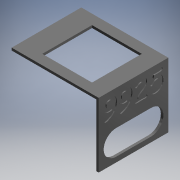
# Autodesk Inventor part: Gen2 Capstone 3D Print 2.0
Saved by Autodesk Inventor 2019 (Build 230136000, 136)
## iProperties
Part Number: Gen2 Capstone 3D Print 2.0
Material: Generic
Document SubType Name: Modeling
Designer: Delta
Appearance: Default
Author: Delta
Autodesk Inventor part; units mm, degrees
ref_plane "YZ Plane" through (0, 0, 0) normal (1, 0, 0) x (0, 1, 0)
ref_plane "XZ Plane" through (0, 0, 0) normal (0, 1, 0) x (-1, 0, 0)
ref_plane "XY Plane" through (0, 0, 0) normal (0, 0, 1) x (1, 0, 0)
sketch "Sketch1" plane through (0, 0, 0) normal (0, 1, 0) x (-1, 0, 0)
  line L0 (0, 0) -> (107.95, 0)
  line L1 (107.95, 0) -> (107.95, -88.9)
  line L2 (107.95, -88.9) -> (0, -88.9)
  line L3 (0, -88.9) -> (0, 0)
  line L4 (81.534, -12.7) -> (18.034, -12.7)
  line L5 (18.034, -12.7) -> (18.034, -76.2)
  line L6 (18.034, -76.2) -> (81.534, -76.2)
  line L7 (81.534, -76.2) -> (81.534, -12.7)
  dimension "d0" = 107.95
  dimension "d1" = 88.9
  dimension "d2" = 63.5
  dimension "d3" = 63.5
  dimension "d4" = 18.034
  dimension "d5" = 12.7
  constraints: 16 end point, 4 parallel, 2 horizontal, 2 perpendicular
  measures "d0" distance of L1.end L2.end
  measures "d1" distance of L0.end L1.end
  measures "d2" distance of L6.end L4.start
  measures "d3" distance of L5.end L6.end
  measures "d4" distance between parallel lines of L3 L5
  measures "d5" distance between parallel lines of L0 L4
extrude "Extrusion1" add sketch "Sketch1" along normal blind 3.175
sketch "Sketch2" plane through (0, 0, 0) normal (1, 0, 0) x (0, 0, -1)
  line L0 (0, 3.175) -> (88.9, 3.175) projected
  line L1 (0, 3.175) -> (88.9, 3.175)
  line L2 (88.9, 3.175) -> (88.9, -79.375)
  line L3 (88.9, -79.375) -> (0, -79.375)
  line L4 (0, -79.375) -> (0, 3.175)
  point P0 (0, 0)
  dimension "d8" = 82.55
  dimension "d9" = 88.9
  dimension "d10" = 88.9
  constraints: 8 end point, 2 parallel, 1 horizontal, 1 perpendicular
  measures "d8" distance of L1.end L2.end
  measures "d9" distance of L0.start L0.end
  measures "d10" distance of L2.end L3.end
extrude "Extrusion2" add sketch "Sketch2" along normal blind 3.175
sketch "Sketch3" plane through (3.175, 0, 0) normal (1, 0, 0) x (0, 0, -1)
  line L0 (4.7988, -3.0029) -> (83.6975, -3.0029) construction
  line L1 (83.6975, -3.0029) -> (83.6975, -35.0341) construction
  line L2 (83.6975, -35.0341) -> (4.7988, -35.0341) construction
  line L3 (4.7988, -35.0341) -> (4.7988, -3.0029) construction
  spline S0 degree 2 poles (17.2249, -18.6506) (16.2825, -18.9793) (14.6827, -19.308) (14.0471, -19.308) knots 0 0 0 1 2 2 2
  spline S1 degree 2 poles (14.0471, -19.308) (10.8913, -19.308) (8.5244, -17.6205) knots 0 0 0 1 1 1
  spline S2 degree 2 poles (8.5244, -17.6205) (5.6316, -15.5386) (5.6316, -11.6814) knots 0 0 0 1 1 1
  spline S3 degree 2 poles (5.6316, -11.6814) (5.6316, -7.2107) (8.5902, -4.9315) knots 0 0 0 1 1 1
  spline S4 degree 2 poles (8.5902, -4.9315) (11.0666, -3.0248) (15.0552, -3.0248) knots 0 0 0 1 1 1
  spline S5 degree 2 poles (15.0552, -3.0248) (18.211, -3.0248) (20.6875, -5.4575) knots 0 0 0 1 1 1
  spline S6 degree 2 poles (20.6875, -5.4575) (23.2735, -7.9996) (23.2954, -11.6157) knots 0 0 0 1 1 1
  spline S7 degree 2 poles (23.2954, -11.6157) (23.3173, -15.5605) (21.7613, -19.2423) knots 0 0 0 1 1 1
  spline S8 degree 2 poles (21.7613, -19.2423) (20.0958, -23.2528) (17.2029, -25.2909) knots 0 0 0 1 1 1
  spline S9 degree 2 poles (17.2029, -25.2909) (15.9976, -26.1456) (13.4116, -27.3291) knots 0 0 0 1 1 1
  spline S10 degree 2 poles (13.4116, -27.3291) (10.453, -28.6659) (9.2257, -28.6659) knots 0 0 0 1 1 1
  spline S11 degree 2 poles (9.2257, -28.6659) (8.3053, -28.6659) (7.6916, -28.0084) knots 0 0 0 1 1 1
  spline S12 degree 2 poles (7.6916, -28.0084) (7.1218, -27.3948) (7.1218, -26.5839) knots 0 0 0 1 1 1
  spline S13 degree 2 poles (7.1218, -26.5839) (7.1218, -25.3128) (8.634, -24.6554) knots 0 0 0 1 1 1
  spline S14 degree 2 poles (8.634, -24.6554) (9.927, -24.239) (11.22, -23.8226) knots 0 0 0 1 1 1
  spline S15 degree 2 poles (11.22, -23.8226) (13.5211, -22.946) (16.151, -20.6887) (17.2249, -18.6506) knots 0 0 0 1 2 2 2
  spline S16 degree 2 poles (14.595, -6.7724) (12.272, -6.7724) (9.9489, -9.0735) (9.927, -11.4185) knots 0 0 0 1 2 2 2
  spline S17 degree 2 poles (9.927, -11.4185) (9.927, -13.3032) (11.3077, -14.3551) knots 0 0 0 1 1 1
  spline S18 degree 2 poles (11.3077, -14.3551) (12.5349, -15.2975) (14.5073, -15.2975) knots 0 0 0 1 1 1
  spline S19 degree 2 poles (14.5073, -15.2975) (15.2963, -15.2975) (17.444, -14.3113) (18.8247, -13.347) knots 0 0 0 1 2 2 2
  spline S20 degree 2 poles (18.8247, -13.347) (18.9781, -12.2512) (18.9781, -11.6157) knots 0 0 0 1 1 1
  spline S21 degree 2 poles (18.9781, -11.6157) (18.9562, -9.972) (17.4878, -8.3503) knots 0 0 0 1 1 1
  spline S22 degree 2 poles (17.4878, -8.3503) (16.0195, -6.7724) (14.595, -6.7724) knots 0 0 0 1 1 1
  spline S23 degree 2 poles (36.883, -18.6506) (35.9406, -18.9793) (34.3408, -19.308) (33.7053, -19.308) knots 0 0 0 1 2 2 2
  spline S24 degree 2 poles (33.7053, -19.308) (30.5494, -19.308) (28.1826, -17.6205) knots 0 0 0 1 1 1
  spline S25 degree 2 poles (28.1826, -17.6205) (25.2897, -15.5386) (25.2897, -11.6814) knots 0 0 0 1 1 1
  spline S26 degree 2 poles (25.2897, -11.6814) (25.2897, -7.2107) (28.2483, -4.9315) knots 0 0 0 1 1 1
  spline S27 degree 2 poles (28.2483, -4.9315) (30.7248, -3.0248) (34.7134, -3.0248) knots 0 0 0 1 1 1
  spline S28 degree 2 poles (34.7134, -3.0248) (37.8692, -3.0248) (40.3456, -5.4575) knots 0 0 0 1 1 1
  spline S29 degree 2 poles (40.3456, -5.4575) (42.9317, -7.9996) (42.9536, -11.6157) knots 0 0 0 1 1 1
  spline S30 degree 2 poles (42.9536, -11.6157) (42.9755, -15.5605) (41.4195, -19.2423) knots 0 0 0 1 1 1
  spline S31 degree 2 poles (41.4195, -19.2423) (39.7539, -23.2528) (36.8611, -25.2909) knots 0 0 0 1 1 1
  spline S32 degree 2 poles (36.8611, -25.2909) (35.6557, -26.1456) (33.0697, -27.3291) knots 0 0 0 1 1 1
  spline S33 degree 2 poles (33.0697, -27.3291) (30.1111, -28.6659) (28.8839, -28.6659) knots 0 0 0 1 1 1
  spline S34 degree 2 poles (28.8839, -28.6659) (27.9634, -28.6659) (27.3498, -28.0084) knots 0 0 0 1 1 1
  spline S35 degree 2 poles (27.3498, -28.0084) (26.78, -27.3948) (26.78, -26.5839) knots 0 0 0 1 1 1
  spline S36 degree 2 poles (26.78, -26.5839) (26.78, -25.3128) (28.2921, -24.6554) knots 0 0 0 1 1 1
  spline S37 degree 2 poles (28.2921, -24.6554) (29.5852, -24.239) (30.8782, -23.8226) knots 0 0 0 1 1 1
  spline S38 degree 2 poles (30.8782, -23.8226) (33.1793, -22.946) (35.8091, -20.6887) (36.883, -18.6506) knots 0 0 0 1 2 2 2
  spline S39 degree 2 poles (34.2532, -6.7724) (31.9301, -6.7724) (29.6071, -9.0735) (29.5852, -11.4185) knots 0 0 0 1 2 2 2
  spline S40 degree 2 poles (29.5852, -11.4185) (29.5852, -13.3032) (30.9658, -14.3551) knots 0 0 0 1 1 1
  spline S41 degree 2 poles (30.9658, -14.3551) (32.1931, -15.2975) (34.1655, -15.2975) knots 0 0 0 1 1 1
  spline S42 degree 2 poles (34.1655, -15.2975) (34.9544, -15.2975) (37.1022, -14.3113) (38.4828, -13.347) knots 0 0 0 1 2 2 2
  spline S43 degree 2 poles (38.4828, -13.347) (38.6362, -12.2512) (38.6362, -11.6157) knots 0 0 0 1 1 1
  spline S44 degree 2 poles (38.6362, -11.6157) (38.6143, -9.972) (37.146, -8.3503) knots 0 0 0 1 1 1
  spline S45 degree 2 poles (37.146, -8.3503) (35.6777, -6.7724) (34.2532, -6.7724) knots 0 0 0 1 1 1
  spline S46 degree 2 poles (59.96, -27.1976) (59.5655, -27.1976) (57.9218, -26.9565) (57.5493, -26.9565) knots 0 0 0 1 2 2 2
  line L4 (57.5493, -26.9565) -> (52.947, -26.9346)
  spline S47 degree 2 poles (52.947, -26.9346) (52.3553, -26.9346) (49.9227, -27.1976) (49.331, -27.1976) knots 0 0 0 1 2 2 2
  spline S48 degree 2 poles (49.331, -27.1976) (49.1557, -27.1976) (48.4982, -27.0661) (48.3229, -27.0661) knots 0 0 0 1 2 2 2
  spline S49 degree 2 poles (48.3229, -27.0661) (46.8984, -27.0661) (46.3943, -25.9265) knots 0 0 0 1 1 1
  spline S50 degree 2 poles (46.3943, -25.9265) (46.0875, -25.2033) (46.0875, -23.6911) knots 0 0 0 1 1 1
  spline S51 degree 2 poles (46.0875, -23.6911) (46.0875, -20.7544) (47.4024, -18.782) knots 0 0 0 1 1 1
  spline S52 degree 2 poles (47.4024, -18.782) (48.3886, -17.2699) (50.6459, -15.7358) knots 0 0 0 1 1 1
  spline S53 degree 2 poles (50.6459, -15.7358) (52.7717, -14.3332) (54.8756, -12.9525) knots 0 0 0 1 1 1
  spline S54 degree 2 poles (54.8756, -12.9525) (57.352, -11.1555) (57.352, -8.8543) knots 0 0 0 1 1 1
  spline S55 degree 2 poles (57.352, -8.8543) (57.352, -8.2626) (55.3796, -7.0792) (54.4373, -7.0792) knots 0 0 0 1 2 2 2
  spline S56 degree 2 poles (54.4373, -7.0792) (52.7717, -7.0792) (49.0461, -10.0597) (48.3448, -10.0597) knots 0 0 0 1 2 2 2
  spline S57 degree 2 poles (48.3448, -10.0597) (47.512, -10.0597) (46.8984, -9.6433) knots 0 0 0 1 1 1
  spline S58 degree 2 poles (46.8984, -9.6433) (46.1094, -9.1392) (46.1094, -8.2407) knots 0 0 0 1 1 1
  spline S59 degree 2 poles (46.1094, -8.2407) (46.1094, -7.2984) (46.8984, -6.5971) knots 0 0 0 1 1 1
  spline S60 degree 2 poles (46.8984, -6.5971) (48.7831, -4.9096) (50.2076, -4.1425) knots 0 0 0 1 1 1
  spline S61 degree 2 poles (50.2076, -4.1425) (52.2457, -3.0248) (54.4373, -3.0248) knots 0 0 0 1 1 1
  spline S62 degree 2 poles (54.4373, -3.0248) (57.1548, -3.0248) (59.3244, -4.4493) knots 0 0 0 1 1 1
  spline S63 degree 2 poles (59.3244, -4.4493) (61.8228, -6.093) (61.8228, -8.7229) knots 0 0 0 1 1 1
  spline S64 degree 2 poles (61.8228, -8.7229) (61.8228, -11.3965) (60.5955, -13.2813) knots 0 0 0 1 1 1
  spline S65 degree 2 poles (60.5955, -13.2813) (59.6531, -14.7715) (57.5712, -16.1741) knots 0 0 0 1 1 1
  spline S66 degree 2 poles (57.5712, -16.1741) (55.6207, -17.4233) (53.6483, -18.6506) knots 0 0 0 1 1 1
  spline S67 degree 2 poles (53.6483, -18.6506) (50.6678, -20.601) (50.4487, -23.0994) knots 0 0 0 1 1 1
  spline S68 degree 2 poles (50.4487, -23.0994) (51.3034, -22.9898) (52.9909, -22.8583) knots 0 0 0 1 1 1
  spline S69 degree 2 poles (52.9909, -22.8583) (56.322, -22.683) (57.7684, -22.683) knots 0 0 0 1 1 1
  spline S70 degree 2 poles (57.7684, -22.683) (59.1272, -22.683) (60.4421, -23.2528) knots 0 0 0 1 1 1
  spline S71 degree 2 poles (60.4421, -23.2528) (62.0638, -23.976) (62.0638, -25.1156) knots 0 0 0 1 1 1
  spline S72 degree 2 poles (62.0638, -25.1156) (62.0638, -25.9265) (61.494, -26.5401) knots 0 0 0 1 1 1
  spline S73 degree 2 poles (61.494, -26.5401) (60.8804, -27.1976) (59.96, -27.1976) knots 0 0 0 1 1 1
  spline S74 degree 2 poles (72.6052, -28.1619) (67.8057, -28.1619) (65.5265, -24.743) knots 0 0 0 1 1 1
  spline S75 degree 2 poles (65.5265, -24.743) (65.132, -24.1294) (65.132, -23.5815) knots 0 0 0 1 1 1
  spline S76 degree 2 poles (65.132, -23.5815) (65.132, -22.7487) (66.4908, -21.5434) (67.3455, -21.5434) knots 0 0 0 1 2 2 2
  spline S77 degree 2 poles (67.3455, -21.5434) (68.2221, -21.5434) (68.8576, -22.2009) knots 0 0 0 1 1 1
  spline S78 degree 2 poles (68.8576, -22.2009) (69.9534, -23.3405) (70.063, -23.4281) knots 0 0 0 1 1 1
  spline S79 degree 2 poles (70.063, -23.4281) (70.9834, -24.0856) (72.6271, -24.0856) knots 0 0 0 1 1 1
  spline S80 degree 2 poles (72.6271, -24.0856) (75.0378, -24.0856) (76.6595, -22.3104) knots 0 0 0 1 1 1
  spline S81 degree 2 poles (76.6595, -22.3104) (78.2155, -20.601) (78.2155, -18.1684) knots 0 0 0 1 1 1
  spline S82 degree 2 poles (78.2155, -18.1684) (78.2155, -15.8235) (76.6595, -13.5004) (75.0816, -13.5004) knots 0 0 0 1 2 2 2
  spline S83 degree 2 poles (75.0816, -13.5004) (72.3203, -13.5004) (70.6328, -15.2975) knots 0 0 0 1 1 1
  spline S84 degree 2 poles (70.6328, -15.2975) (69.9753, -16.0426) (69.2959, -16.7877) knots 0 0 0 1 1 1
  spline S85 degree 2 poles (69.2959, -16.7877) (68.4412, -17.5767) (67.4989, -17.5767) knots 0 0 0 1 1 1
  spline S86 degree 2 poles (67.4989, -17.5767) (66.6003, -17.5767) (65.3512, -16.3494) (65.3512, -15.5166) knots 0 0 0 1 2 2 2
  spline S87 degree 2 poles (65.3512, -15.5166) (65.3512, -15.166) (65.6142, -12.7772) knots 0 0 0 1 1 1
  spline S88 degree 2 poles (65.6142, -12.7772) (66.1401, -8.175) (66.1401, -6.6628) knots 0 0 0 1 1 1
  spline S89 degree 2 poles (66.1401, -6.6628) (66.1401, -6.2683) (65.5922, -4.9534) (65.5922, -4.5808) knots 0 0 0 1 2 2 2
  spline S90 degree 2 poles (65.5922, -4.5808) (65.5922, -3.7919) (66.4031, -3.3755) knots 0 0 0 1 1 1
  spline S91 degree 2 poles (66.4031, -3.3755) (67.0167, -3.0687) (67.8714, -3.0687) knots 0 0 0 1 1 1
  spline S92 degree 2 poles (67.8714, -3.0687) (68.1783, -3.0687) (69.4494, -3.1782) (69.7781, -3.1782) knots 0 0 0 1 2 2 2
  line L5 (69.7781, -3.1782) -> (77.3389, -3.2002)
  spline S93 degree 2 poles (77.3389, -3.2002) (77.6238, -3.2002) (79.4647, -3.0029) (79.7715, -3.0029) knots 0 0 0 1 2 2 2
  spline S94 degree 2 poles (79.7715, -3.0029) (80.6262, -3.0029) (81.722, -4.0987) (81.722, -4.9315) knots 0 0 0 1 2 2 2
  spline S95 degree 2 poles (81.722, -4.9315) (81.722, -7.2764) (76.9444, -7.2764) knots 0 0 0 1 1 1
  spline S96 degree 2 poles (76.9444, -7.2764) (76.5719, -7.2764) (75.4323, -7.2545) (75.235, -7.2545) knots 0 0 0 1 2 2 2
  line L6 (75.235, -7.2545) -> (70.5451, -7.2545)
  spline S97 degree 2 poles (70.5451, -7.2545) (70.5013, -8.2188) (70.1506, -10.4323) knots 0 0 0 1 1 1
  spline S98 degree 2 poles (70.1506, -10.4323) (72.2107, -9.4241) (75.0816, -9.4241) knots 0 0 0 1 1 1
  spline S99 degree 2 poles (75.0816, -9.4241) (78.8949, -9.4241) (80.8892, -12.2732) knots 0 0 0 1 1 1
  spline S100 degree 2 poles (80.8892, -12.2732) (82.5329, -14.6181) (82.5329, -18.1684) knots 0 0 0 1 1 1
  spline S101 degree 2 poles (82.5329, -18.1684) (82.5329, -22.4419) (79.903, -25.2471) knots 0 0 0 1 1 1
  spline S102 degree 2 poles (79.903, -25.2471) (77.1417, -28.1619) (72.6052, -28.1619) knots 0 0 0 1 1 1
  point P0 (0, 0)
  constraints: 2 other
extrude "Extrusion3" cut sketch "Sketch3" against normal blind 1.27
sketch "Sketch4" plane through (3.175, 0, 0) normal (1, 0, 0) x (0, 0, -1)
  line L0 (6.35, -73.025) -> (82.55, -73.025)
  line L1 (82.55, -73.025) -> (82.55, -41.275)
  line L2 (82.55, -41.275) -> (6.35, -41.275)
  line L3 (6.35, -41.275) -> (6.35, -73.025)
  line L4 (88.9, 3.175) -> (0, 3.175) projected
  line L5 (61.9766, -27.1976) -> (61.9766, -27.0661) projected
  line L6 (48.3229, -28.9381) -> (46.3943, -28.9381) projected
  line L7 (46.3126, -3.0248) -> (46.3126, -4.4493) projected
  line L8 (52.9909, -8.1488) -> (57.7684, -8.1488) projected
  line L9 (46.8478, -22.683) -> (46.8478, -23.2528) projected
  line L10 (52.947, -25.9947) -> (49.331, -25.9947) projected
  line L11 (28.7549, -23.8226) -> (28.7549, -18.6506) projected
  line L12 (36.883, -25.8094) -> (33.7053, -25.8094) projected
  line L13 (9.6946, -23.8226) -> (9.6946, -18.6506) projected
  line L14 (17.2249, -25.8094) -> (14.0471, -25.8094) projected
  line L15 (65.6405, -17.5767) -> (65.6405, -15.5166) projected
  line L16 (65.3512, -24.4303) -> (65.6142, -24.4303) projected
  line L17 (66.6902, -3.0029) -> (66.6902, -4.9315) projected
  line L18 (81.722, -3.5381) -> (76.9444, -3.5381) projected
  line L19 (80.6252, -7.2764) -> (80.6252, -7.2545) projected
  line L20 (75.235, -7.2545) -> (70.5451, -7.2545) projected
  line L21 (69.963, -7.2545) -> (69.963, -10.4323) projected
  line L22 (88.9, 3.175) -> (0, 3.175) projected
  line L23 (0, 3.175) -> (0, -79.375) projected
  line L24 (0, -79.375) -> (88.9, -79.375) projected
  line L25 (88.9, -79.375) -> (88.9, 3.175) projected
  line L26 (28.2921, -24.6554) -> (30.8782, -23.8226) projected
  line L27 (8.634, -24.6554) -> (11.22, -23.8226) projected
  point P0 (0, 0)
  point P1 (49.331, -27.1976)
  point P2 (48.3229, -27.0661)
  point P3 (57.7684, -22.683)
  point P4 (36.883, -18.6506)
  point P5 (17.2249, -18.6506)
  point P6 (65.3512, -15.5166)
  point P7 (81.722, -4.9315)
  point P8 (76.9444, -7.2764)
  dimension "d15" = 76.2
  dimension "d16" = 31.75
  dimension "d17" = 88.9
  dimension "d18" = 6.35
  dimension "d19" = 6.35
  constraints: 8 end point, 2 parallel, 1 horizontal, 1 perpendicular, 73 other
  measures "d15" distance of L1.end L2.end
  measures "d16" distance of L0.end L1.end
  measures "d17" distance of L23.end L24.end
  measures "d18" distance between parallel lines of L24 L0
  measures "d19" distance between parallel lines of L23 L3
extrude "Extrusion4" cut sketch "Sketch4" against normal through all contours L3 L2 L1 L0
fillet "Fillet1" radius 15.875 4 edges at (1.5875, -73.025, -82.55) (1.5875, -73.025, -6.35) (1.5875, -41.275, -6.35) (1.5875, -41.275, -82.55)
equation "\"d5\" = -0.5 * d2 + 0.5 * d1"
equation "\"d10\" = d9"
equation "\"d19\" = -0.5 * d15 + 0.5 * d17"
body "Solid1"
